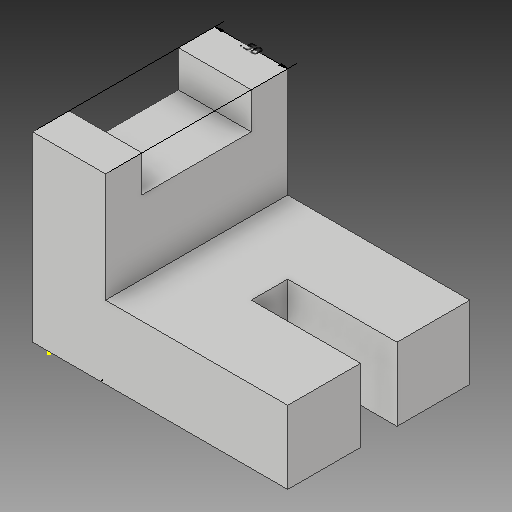
# Autodesk Inventor part: arthurWeiActivity 7.1#1
Saved by Autodesk Inventor 2018 (Build 220112000, 112)
## iProperties
Created: 2019-01-14
Part Number: arthurWeiActivity 7.1#1
Material: Generic
Document SubType Name: Modeling
Designer: This kid
Density: 1 g/cm^3
Appearance: Default
Author: This kid
Autodesk Inventor part; units mm, degrees
ref_plane "YZ Plane" through (0, 0, 0) normal (1, 0, 0) x (0, 1, 0)
ref_plane "XZ Plane" through (0, 0, 0) normal (0, 1, 0) x (-1, 0, 0)
ref_plane "XY Plane" through (0, 0, 0) normal (0, 0, 1) x (1, 0, 0)
sketch "Sketch1" plane through (0, 0, 0) normal (0, 0, 1) x (1, 0, 0)
  line L0 (-2.83, 31.9472) -> (9.87, 31.9472)
  line L1 (9.87, 31.9472) -> (9.87, 12.8972)
  line L2 (9.87, 0.1972) -> (-2.83, 0.1972)
  line L3 (-2.83, 0.1972) -> (-2.83, 31.9472)
  line L4 (9.87, 12.8972) -> (9.8204, 12.9735)
  line L5 (9.87, 0.1972) -> (41.62, 0.1972)
  line L6 (41.62, 0.1972) -> (41.62, 12.8972)
  line L7 (41.62, 12.8972) -> (9.87, 12.8972)
  point P0 (0, 0)
  dimension "d0" = 12.7
  dimension "d1" = 31.75
  dimension "d4" = 31.75
  dimension "d5" = 12.7
  dimension "d6" = 12.7
  dimension "d17" = 44.45
  constraints: 16 end point, 3 parallel, 2 horizontal, 2 perpendicular
  measures "d0" distance of L2.start L2.end
  measures "d1" distance of L0.end L2.start
  measures "d4" distance of L1.end L6.end
  measures "d5" distance of L6.end L5.end
  measures "d6" distance of L0.start L0.end
  measures "d17" distance of L5.end L2.end
extrude "Extrusion1" add sketch "Sketch1" along normal blind 31.75
sketch "Sketch2" plane through (41.62, 0.1972, 0) normal (1, 0, 0) x (0, 0, -1)
  line L0 (-31.75, 0) -> (-31.75, 12.7) projected
  line L1 (-31.75, 12.7) -> (-15.875, 12.7)
  line L2 (0, 12.7) -> (-31.75, 12.7) projected
  line L3 (0, 0) -> (-31.75, 0) projected
  line L4 (-12.7, 12.7) -> (-19.05, 12.7)
  line L5 (-19.05, 12.7) -> (-19.05, 0)
  line L6 (-19.05, 0) -> (-12.7, 0)
  line L7 (-12.7, 0) -> (-12.7, 12.7)
  point P0 (0, -0.1972)
  dimension "d11" = 15.875
  dimension "d13" = 6.35
  dimension "d14" = 3.175
  constraints: 10 end point, 2 parallel, 2 point on line, 1 horizontal, 1 midpoint, 1 perpendicular
  measures "d11" distance of L0.end L1.end
  measures "d13" distance of L6.end L5.end
  measures "d14" distance of L1.end L4.start
extrude "Extrusion2" cut sketch "Sketch2" against normal blind 19.05 contours L5 L1 L2 L7 L3
sketch "Sketch3" plane through (9.87, 12.8972, 0) normal (1, 0, 0) x (0, 0, -1)
  line L0 (-31.75, 19.05) -> (-25.4, 19.05)
  line L1 (0, 19.05) -> (-31.75, 19.05) projected
  line L2 (0, 19.05) -> (-6.35, 19.05)
  line L3 (-25.4, 19.05) -> (-6.35, 19.05)
  line L4 (-6.35, 19.05) -> (-6.35, 12.7)
  line L5 (-6.35, 12.7) -> (-25.4, 12.7)
  line L6 (-25.4, 12.7) -> (-25.4, 19.05)
  point P0 (0, -12.8972)
  dimension "d18" = 6.35
  dimension "d19" = 6.35
  dimension "d20" = 6.35
  constraints: 12 end point, 2 parallel, 2 point on line, 1 horizontal, 1 perpendicular
  measures "d18" distance of L0.start L0.end
  measures "d19" distance of L1.start L2.end
  measures "d20" distance of L3.end L4.end
extrude "Extrusion3" cut sketch "Sketch3" against normal through all
sketch "Sketch4" plane through (0, 0, 31.75) normal (0, 0, 1) x (1, 0, 0)
  point P0 (0, 0)
body "Solid1"
